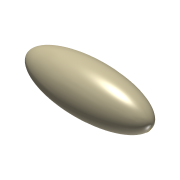
# Autodesk Inventor part: Flyspresso-CAD-files:24W EMBRYO EXAMPLE
Saved by Autodesk Inventor 2015 SP1 (Build 190203100, 203)
## iProperties
Created: 2016-01-19
Material: Generic
Vendor: HHMI: JRC - ID&F
Document SubType Name: Modeling
Designer: JORDANJ
Density: 1 g/cm^3
Appearance: Fine - Cream
RuleStatus: InUse
AfterDocSave0: file://Part Number Cleaner
DESIGN DEPARTMENT: HHMI: JRC - ID&F
ALTERED ITEM PART NUMBER: N/A
ALTERED ITEM VENDOR: N/A
ALTERED ITEM DESCRIPTION: N/A
Author: JORDANJ
Revision Number: 0
Autodesk Inventor part; units mm, degrees
ref_plane "YZ Plane" through (0, 0, 0) normal (1, 0, 0) x (0, 1, 0)
ref_plane "XZ Plane" through (0, 0, 0) normal (0, 1, 0) x (-1, 0, 0)
ref_plane "XY Plane" through (0, 0, 0) normal (0, 0, 1) x (1, 0, 0)
sketch "Sketch1" plane through (0, 0, 0) normal (0, 0, 1) x (1, 0, 0)
  line L0 (-0.255, 0.09) -> (0.255, 0.09)
  ellipse E0 centre (0, 0.09) end of major axis (-0.255, 0.09) minor radius 0.09 (-0.255, 0.09) -> (0.255, 0.09) ccw
  ellipse E1 centre (0, 0.09) end of major axis (-0.255, 0.09) minor radius 0.09 (0.255, 0.09) -> (-0.255, 0.09) ccw
  point P0 (0, 0)
  point P1 (0, 0.09)
  dimension "d2" = 0.09
  dimension "d1" = 0.51
  constraints: 2 end point, 1 coincident, 1 horizontal, 1 midpoint, 1 vertical alignment, 9 other
  measures "d1" distance of L0.start L0.end
revolve "Revolution1" add sketch "Sketch1" angle 360 about axis through (-0.255, 0.09, 0) along (1, 0, 0) contours L0 E0
body "Solid1"
